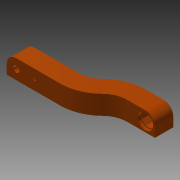
# Autodesk Inventor part: xy forearm
Saved by Autodesk Inventor 2013 (Build 170138000, 138)
## iProperties
Created: 2014-02-19
Part Number: xy forearm
Material: Generic
Document SubType Name: Modeling
Designer: employee
Density: 1 g/cm^3
Author: employee
Autodesk Inventor part; units mm, degrees
ref_plane "YZ Plane" through (0, 0, 0) normal (1, 0, 0) x (0, 1, 0)
ref_plane "XZ Plane" through (0, 0, 0) normal (0, 1, 0) x (-1, 0, 0)
ref_plane "XY Plane" through (0, 0, 0) normal (0, 0, 1) x (1, 0, 0)
sketch "Sketch1" plane through (0, 0, 0) normal (0, 0, 1) x (1, 0, 0)
  line L0 (0, 0) -> (60, 0)
  arc A0 (60, 0) -> (101.2397, 16.8131) centre (60, 58.9835) ccw
  arc A1 (125, 26.5) -> (101.2397, 16.8131) centre (125, -7.4835) ccw
  line L1 (125, 26.5) -> (150, 26.5)
  line L2 (150, 26.5) -> (150, 51.5)
  line L3 (150, 51.5) -> (125, 51.5)
  arc A2 (125, 51.5) -> (83.7603, 34.6869) centre (125, -7.4835) ccw
  arc A3 (60, 25) -> (83.7603, 34.6869) centre (60, 58.9835) ccw
  line L4 (60, 25) -> (0, 25)
  line L5 (0, 25) -> (0, 0)
  dimension "d0" = 25
  dimension "d1" = 60
  dimension "d2" = 25
  dimension "d3" = 150
  dimension "d4" = 1.5
  constraints: 12 end point, 8 point on circle, 6 tangent, 5 parallel, 4 centre point, 1 coincident, 1 concentric, 1 equal radius, 1 horizontal, 1 perpendicular
  measures "d0" distance of L4.end L0.start
  measures "d1" distance of L0.start L0.end
  measures "d2" distance of L2.end L3.end
  measures "d3" distance between parallel lines of L5 L2
  measures "d4" distance between parallel lines of L4 L1
extrude "Extrusion1" add sketch "Sketch1" along normal blind 26
sketch "Sketch2" plane through (125, 26.5, 0) normal (0, -1, 0) x (1, 0, 0)
  line L0 (25, 0) -> (25, 26) projected
  circle A0 centre (25, 13) radius 13
  point P0 (-125, 0)
  constraints: 1 midpoint, 1 vertical alignment, 2 other
extrude "Extrusion2" add sketch "Sketch2" against normal up to surface (25 mm away)
sketch "Sketch3" plane through (0, 0, 0) normal (0, -1, 0) x (1, 0, 0)
  line L0 (0, 0) -> (0, 26) projected
  circle A0 centre (0, 13) radius 13
  line L1 (0, 0) -> (-13, 0)
  line L2 (-13, 0) -> (-13, 13)
  constraints: 4 end point, 2 point on circle, 2 tangent, 1 centre point, 1 midpoint, 1 perpendicular, 1 vertical
extrude "Extrusion3" add sketch "Sketch3" against normal up to surface (25 mm away)
sketch "Sketch4" plane through (125, 26.5, 0) normal (0, -1, 0) x (1, 0, 0)
  line L0 (0, 0) -> (25, 0) projected
  arc A0 (25, 0) -> (25, 26) centre (25, 13) ccw projected
  line L1 (25, 0) -> (38, 0)
  line L2 (38, 0) -> (38, 13)
  point P0 (-125, 0)
  constraints: 4 end point, 1 collinear, 1 point on circle, 1 tangent, 1 vertical
extrude "Extrusion4" add sketch "Sketch4" against normal up to surface (25 mm away)
sketch "Sketch5" plane through (60, 0, 0) normal (0, -1, 0) x (1, 0, 0)
  arc A0 (-60, 26) -> (-73, 13) centre (-60, 13) ccw projected
  circle A1 centre (-60, 13) radius 4.1
  point P0 (-60, 0)
  dimension "d13" = 8.2
  constraints: 1 centre point, 1 coincident
  measures "d13" diameter of A1
extrude "Extrusion5" cut sketch "Sketch5" against normal through all
sketch "Sketch6" plane through (60, 0, 0) normal (0, -1, 0) x (1, 0, 0)
  arc A0 (-60, 26) -> (-73, 13) centre (-60, 13) ccw projected
  line L0 (-73, 13) -> (-73, 0) projected
  line L1 (-60, 13) -> (-35, 13)
  circle A1 centre (-35, 13) radius 1.5
  point P0 (-60, 0)
  dimension "d17" = 3
  dimension "d19" = 25
  constraints: 2 end point, 1 centre point, 1 coincident, 1 perpendicular
  measures "d17" diameter of A1
  measures "d19" distance of L1.start L1.end
extrude "Extrusion6" cut sketch "Sketch6" against normal through all
sketch "Sketch7" plane through (125, 26.5, 0) normal (0, -1, 0) x (1, 0, 0)
  arc A0 (38, 13) -> (25, 26) centre (25, 13) ccw projected
  circle A1 centre (25, 13) radius 10.5 construction
  circle A2 centre (25, 13) radius 7.5 construction
  line L0 (21.2721, 22) -> (28.7279, 22)
  line L1 (28.7279, 22) -> (34, 16.7279)
  line L2 (34, 16.7279) -> (34, 9.2721)
  line L3 (34, 9.2721) -> (28.7279, 4)
  line L4 (28.7279, 4) -> (21.2721, 4)
  line L5 (21.2721, 4) -> (16, 9.2721)
  line L6 (16, 9.2721) -> (16, 16.7279)
  line L7 (16, 16.7279) -> (21.2721, 22)
  point P0 (-125, 0)
  dimension "d22" = 21
  dimension "d24" = 15
  dimension "d25" = 18
  constraints: 16 end point, 3 coincident, 2 centre point, 1 horizontal, 17 other
  measures "d22" diameter of A1
  measures "d24" diameter of A2
  measures "d25" distance between parallel lines of L4 L0
extrude "Extrusion7" cut sketch "Sketch7" against normal through all
sketch "Sketch8" plane through (125, 26.5, 0) normal (0, -1, 0) x (1, 0, 0)
  line L0 (16, 16.7279) -> (21.2721, 22) projected
  line L1 (21.2721, 22) -> (28.7279, 22) projected
  line L2 (28.7279, 22) -> (34, 16.7279) projected
  line L3 (34, 16.7279) -> (34, 9.2721) projected
  line L4 (34, 9.2721) -> (28.7279, 4) projected
  line L5 (28.7279, 4) -> (21.2721, 4) projected
  line L6 (21.2721, 4) -> (16, 9.2721) projected
  line L7 (16, 9.2721) -> (16, 16.7279) projected
  arc A0 (38, 13) -> (25, 26) centre (25, 13) ccw projected
  circle A1 centre (25, 13) radius 10.55
  point P0 (-125, 0)
  dimension "d28" = 21.1
  constraints: 1 centre point, 1 coincident
  measures "d28" diameter of A1
extrude "Extrusion8" cut sketch "Sketch8" against normal blind 4
sketch "Sketch9" plane through (125, 51.5, 26) normal (0, 1, 0) x (1, 0, 0)
  line L0 (21.2721, 4) -> (16, 9.2721) projected
  line L1 (16, 9.2721) -> (16, 16.7279) projected
  line L2 (16, 16.7279) -> (21.2721, 22) projected
  line L3 (21.2721, 22) -> (28.7279, 22) projected
  line L4 (28.7279, 22) -> (34, 16.7279) projected
  line L5 (34, 16.7279) -> (34, 9.2721) projected
  line L6 (34, 9.2721) -> (28.7279, 4) projected
  line L7 (28.7279, 4) -> (21.2721, 4) projected
  circle A0 centre (25, 13) radius 10.55 projected
  point P0 (-125, 26)
extrude "Extrusion9" cut sketch "Sketch9" against normal blind 4
body "Solid1"
